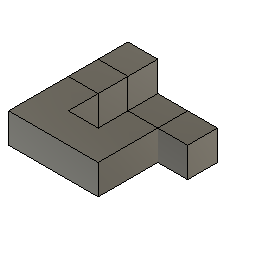
BooleanIntersectMultiTool (Autodesk Fusion 360 design; units mm, degrees)
Autodesk Fusion 360 part; units mm, degrees
sketch "Sketch1" plane through (0, 0, 0) normal (0, 0, 1) x (1, 0, 0)
  line L0 (0, 0) -> (-30, 0)
  line L1 (-30, 0) -> (-30, 10)
  line L2 (-30, 10) -> (0, 10)
  line L3 (0, 10) -> (0, 0)
  line L4 (-30, 10) -> (-20, 10)
  line L5 (-20, 10) -> (-20, 30)
  line L6 (-20, 30) -> (-30, 30)
  line L7 (-30, 30) -> (-30, 10)
  line L8 (0, 10) -> (-10, 10)
  line L9 (-10, 10) -> (-10, 30)
  line L10 (-10, 30) -> (0, 30)
  line L11 (0, 30) -> (0, 10)
  line L12 (-30, 30) -> (0, 30)
  line L13 (0, 30) -> (0, 20)
  line L14 (0, 20) -> (-30, 20)
  line L15 (-30, 20) -> (-30, 30)
  line L16 (-20, 30) -> (-30, 30)
  line L17 (-30, 30) -> (-30, 40)
  line L18 (-30, 40) -> (-20, 40)
  line L19 (-20, 40) -> (-20, 30)
  line L20 (0, 30) -> (10, 30)
  line L21 (10, 30) -> (10, 20)
  line L22 (10, 20) -> (0, 20)
  line L23 (0, 20) -> (0, 30)
  constraint horizontal L0
  constraint vertical L1
  constraint horizontal L2
  constraint vertical L3
  constraint coincident L0.start L3.end
  constraint horizontal L4
  constraint vertical L5
  constraint horizontal L6
  constraint vertical L7
  constraint horizontal L8
  constraint vertical L9
  constraint horizontal L10
  constraint vertical L11
  constraint horizontal L12
  constraint vertical L13
  constraint horizontal L14
  constraint vertical L15
  constraint midpoint L11 L13.end
  constraint horizontal L16
  constraint vertical L17
  constraint horizontal L18
  constraint vertical L19
  constraint horizontal L20
  constraint vertical L21
  constraint horizontal L22
  constraint vertical L23
extrude "Extrude1" add sketch "Sketch1" along normal blind 10 contours L0 L1 L2 L3 L4 L8 | L2 L8 L9 L11 L14 | L2 L4 L5 L7 L14 | L9 L10 L11 L12 L13 L14 L23 | L5 L6 L7 L12 L14 L15 L16 makes body 1
extrude "Extrude2" add sketch "Sketch1" along normal blind 10 separate body contours L9 L10 L11 L12 L13 L14 L23 | L11 L13 L20 L21 L22 L23 | L5 L6 L7 L12 L14 L15 L16 | L6 L12 L16 L17 L18 L19 makes body 2 at (-3.3333, 23.3333, 0) makes body 3 at (-26.6667, 26.6667, 0) in component "Tool"
component "Tool" placed x (1, 0, 0) y (0, 1, 0) z (0, 0, 1) at (0, 0, 0)
